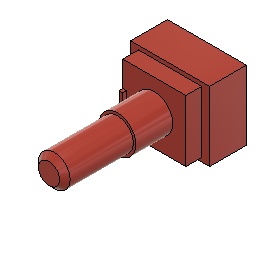
Encoder (Autodesk Fusion 360 design; units mm, degrees)
Autodesk Fusion 360 part; units mm, degrees
sketch "Sketch1" plane through (0, 0, 0) normal (0, 0, 1) x (1, 0, 0)
  line L0 (6, -5.85) -> (-6, -5.85)
  line L1 (-6, -5.85) -> (-6, 5.85)
  line L2 (-6, 5.85) -> (6, 5.85)
  line L3 (6, 5.85) -> (6, -5.85)
  line L4 (6, -5.85) -> (-6, 5.85) construction
  line L5 (-6, -5.85) -> (6, 5.85) construction
  circle A0 centre (0, 0) radius 3.5
  circle A1 centre (0, 0) radius 3
  line L6 (-6, 1) -> (-5.3, 1)
  line L7 (-5.3, 1) -> (-5.3, -1)
  line L8 (-5.3, -1) -> (-6, -1)
  line L9 (-6, -1) -> (-6, 1)
  line L10 (-7.5, -6.6) -> (7.5, -6.6)
  line L11 (7.5, -6.6) -> (7.5, 6.6)
  line L12 (7.5, 6.6) -> (-7.5, 6.6)
  line L13 (-7.5, 6.6) -> (-7.5, -6.6)
  line L14 (-7.5, -6.6) -> (7.5, 6.6) construction
  line L15 (7.5, -6.6) -> (-7.5, 6.6) construction
  point P0 (-6, 0)
  point P1 (-6, 0)
  dimension "d77" = 12
  dimension "d78" = 11.7
  dimension "d79" = 7
  dimension "d80" = 6
  dimension "d81" = 0.7
  dimension "d82" = 2
  dimension "d83" = 15
  dimension "d84" = 13.2
  dimension "d260" = 0
  dimension "d261" = 0
  dimension "d262" = 0
  dimension "d263" = 0
  constraint perpendicular L0 L1
  constraint parallel L0 L2
  constraint parallel L1 L3
  constraint horizontal L0
  constraint coincident L4 A0.centre
  constraint coincident L5 A0.centre
  constraint coincident A0.centre A1.centre
  constraint midpoint L1 P1
  constraint horizontal L6
  constraint vertical L7
  constraint horizontal L8
  constraint vertical L9
  constraint midpoint L9 P1
  constraint coincident P1 P0
  constraint perpendicular L10 L11
  constraint parallel L10 L12
  constraint parallel L11 L13
  constraint horizontal L10
  constraint coincident L14 A0.centre
  constraint coincident L15 A0.centre
  measures "d77" distance of L0.start L0.end
  measures "d78" distance of L0.end L1.end
  measures "d79" diameter of A0
  measures "d80" diameter of A1
  measures "d81" distance of L6.start L6.end
  measures "d82" distance of L6.end L7.end
  measures "d83" distance of L11.end L12.end
  measures "d84" distance of L10.end L11.end
extrude "Extrude1" add sketch "Sketch1" along normal blind 7 contours A0 | A1 makes body 1
extrude "Extrude2" add sketch "Sketch1" along normal blind 20 contours A1 bodies 1
chamfer "Chamfer1" distance 1 angle 45 1 edges at (-2.797, -1.0848, 20) on bodies 1
extrude "Extrude3" add sketch "Sketch1" against normal blind 6.5 separate body contours L0 L1 L2 L3 L6 L7 L8 | L1 L6 L7 L8 L9 makes body 2
extrude "Extrude4" add sketch "Sketch1" against normal blind 7 from surface at -3 contours L10 L11 L12 L13 bodies 2
extrude "Extrude5" add sketch "Sketch1" along normal blind 0.7 contours L1 L6 L7 L8 L9 bodies 2
combine "Combine1" operation add target body 2 tool bodies 1
named bodies: "Encoder"
